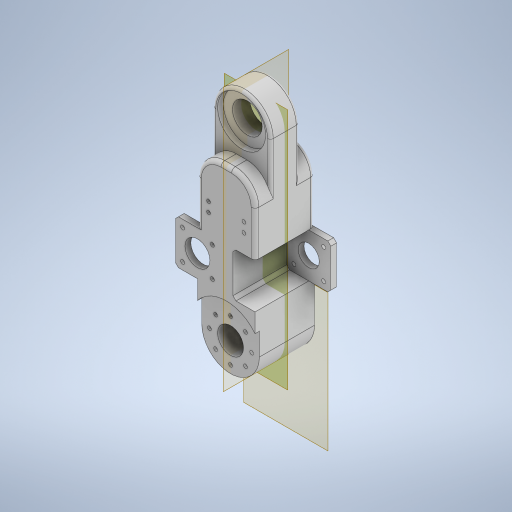
# Autodesk Inventor part: lower arm
Saved by Autodesk Inventor 2024 (Build 280153000, 153)
## iProperties
Created: 2024-02-21
Part Number: lower arm
Material: Generic
Document SubType Name: Modeling
Designer: MaartenGeorgesBuelen
Density: 1 g/cm^3
Appearance: Default
Author: MaartenGeorgesBuelen
## iProperties of the stored document lower arm_3DPrint.ipt
Created: 2024-02-21
Part Number: lower arm_3DPrint
Material: Generic
Document SubType Name: Modeling
Designer: MaartenGeorgesBuelen
Density: 1 g/cm^3
Appearance: Default
Author: MaartenGeorgesBuelen
Autodesk Inventor part; units mm, degrees
ref_plane "YZ Plane" through (0, 0, 0) normal (1, 0, 0) x (0, 1, 0)
ref_plane "XZ Plane" through (0, 0, 0) normal (0, 1, 0) x (-1, 0, 0)
ref_plane "Work Plane1" through (0, 0, 0) normal (0, 0, 1) x (1, 0, 0)
sketch "main" plane through (0, 0, 0) normal (0, 0, 1) x (1, 0, 0)
  circle A0 centre (35, 100) radius 13.5 projected
  arc A1 (31.5, 130) -> (0, 98.5) centre (31.5, 98.5) ccw projected
  line L0 (31.5, 130) -> (38.5, 130) projected
  arc A2 (70, 98.5) -> (38.5, 130) centre (38.5, 98.5) ccw projected
  circle A3 centre (35, 100) radius 30
  line L1 (5, 100) -> (65, 100)
  line L2 (65, 100) -> (65, 260)
  line L3 (65, 260) -> (5, 260)
  line L4 (5, 260) -> (5, 100)
  line L5 (55, 260) -> (15, 260)
  point P0 (0, 0)
  point P1 (0.0085, 99.2302)
  point P2 (69.9915, 99.2302)
  point P3 (35, 70)
  point P4 (48.5, 100)
  point P5 (21.5, 100)
  dimension "d0" = 60
  dimension "d4" = 160
  dimension "d5" = 60
  dimension "d6" = 30
  constraints: 10 end point, 2 horizontal, 2 parallel, 2 point on circle, 1 centre point, 1 coincident, 1 perpendicular, 1 point on line
  measures "d0" diameter of A3
  measures "d4" distance of L2.end L1.end
  measures "d5" distance of L2.end L3.end
  measures "d6" distance from line of A3.centre L4
ref_plane "Work Plane2" through (0, 68.4, 62) normal (0, 0, -1) x (0, 1, 0)
extrude "main extrude" add sketch "main" along normal up to surface (62 mm away) contours L1 A3 A0 | A0 L1 A3 | A3 L0 A2 L2 | L4 A1 L0 A3 | L0 A1 L4 L3 L2 A2
ref_plane "midplane" through (0, 0, 31) normal (0, 0, -1) x (-1, 0, 0)
mirror "right motor" about plane through (0, 0, 31) normal (0, 0, -1)
sketch "Sketch7" plane through (35, 100, 62) normal (0, 0, 1) x (1, 0, 0)
  circle A0 centre (-15.5563, 15.5563) radius 2
  circle A1 centre (0, 22) radius 2
  circle A2 centre (15.5563, 15.5563) radius 2
  circle A3 centre (22, 0) radius 2
  circle A4 centre (15.5563, -15.5563) radius 2
  circle A5 centre (0, -22) radius 2
  circle A6 centre (-15.5563, -15.5563) radius 2
  circle A7 centre (-22, 0) radius 2
  point P0 (-35, -100)
  constraints: 8 centre point, 16 other
extrude "screwholes" cut sketch "Sketch7" against normal blind 10
sketch "Sketch8" plane through (65, 100, 0) normal (1, 0, 0) x (0, 0, -1)
  line L0 (-62, 0) -> (-62, 160) projected
  line L1 (0, 0) -> (-62, 0) projected
  line L2 (0, 0) -> (0, 160) projected
  line L3 (0, 160) -> (-62, 160) projected
  line L4 (-31, 160) -> (-16, 160)
  line L5 (-16, 160) -> (-16, 220)
  line L6 (-16, 220) -> (-31, 220)
  line L7 (-31, 220) -> (-31, 160)
  line L8 (-31, 220) -> (-46, 220)
  line L9 (-46, 220) -> (-46, 160)
  line L10 (-46, 160) -> (-31, 160)
  line L11 (-31, 160) -> (-31, 220)
  point P0 (0, -100)
  point P1 (-46, 160)
  dimension "d39" = 15
  dimension "d40" = 60
  dimension "d41" = 15
  constraints: 16 end point, 5 parallel, 2 horizontal, 2 perpendicular, 1 midpoint
  measures "d39" distance of L6.end L5.end
  measures "d40" distance of L5.end L4.end
  measures "d41" distance of L10.end L9.end
extrude "arm joint" add sketch "Sketch8" against normal up to surface (60 mm away) contours L9 L8 L7 L3 | L7 L6 L5 L3
sketch "Sketch10" plane through (65, 260, 16) normal (0, 0, -1) x (-1, 0, 0)
  line L0 (60, 0) -> (60, 60) projected
  line L1 (0, 60) -> (60, 60) projected
  line L2 (0, 0) -> (0, 60) projected
  line L3 (60, 0) -> (0, 0) projected
  circle A0 centre (30, 32.1294) radius 19
  circle A1 centre (30, 32.1294) radius 13.5
  circle A2 centre (30, 32.1294) radius 25
  point P0 (65, -260)
  dimension "d93" = 4.2
  dimension "d45" = 38
  dimension "d46" = 27
  dimension "d47" = 6
  constraints: 3 centre point, 1 coincident
  measures "d45" diameter of A0
  measures "d46" diameter of A1
  measures "d47" radial gap between concentric circles of A0 A2
extrude "bearing hole" cut sketch "Sketch10" against normal blind 6 contours A0 | A1 | A2
sketch "Sketch11" plane through (35, 292.1294, 22) normal (0, 0, -1) x (-1, 0, 0)
  circle A0 centre (0, 0) radius 25 projected
  circle A1 centre (0, 0) radius 13.5
  point P0 (35, -292.1294)
  dimension "d50" = 27
  constraints: 1 centre point, 1 coincident
  measures "d50" diameter of A1
extrude "axle hole" cut sketch "Sketch11" against normal through all contours A1
mirror "Mirror3" about plane through (0, 0, 31) normal (0, 0, -1) of "bearing hole"
fillet "Fillet1" radius 30 2 edges at (65, 320, 31) (5, 320, 31)
fillet "Fillet3" radius 24.5 2 edges at (5, 260, 54) (65, 260, 54)
mirror "Mirror4" about plane through (0, 0, 31) normal (0, 0, -1) of "Fillet3"
sketch "Sketch14" plane through (35, 100, 62) normal (0, 0, 1) x (1, 0, 0)
  line L0 (9, 85) -> (11, 87) projected
  line L1 (9, 47) -> (9, 85) projected
  line L2 (11, 45) -> (9, 47) projected
  line L3 (49, 45) -> (11, 45) projected
  line L4 (51, 47) -> (49, 45) projected
  line L5 (51, 85) -> (51, 47) projected
  line L6 (49, 87) -> (51, 85) projected
  line L7 (11, 87) -> (49, 87) projected
  line L8 (49.8284, 89) -> (53, 85.8284)
  line L9 (53, 85.8284) -> (53, 46.1716)
  line L10 (53, 46.1716) -> (49.8284, 43)
  line L11 (49.8284, 43) -> (10.1716, 43)
  line L12 (10.1716, 43) -> (7, 46.1716)
  line L13 (7, 46.1716) -> (7, 85.8284)
  line L14 (7, 85.8284) -> (10.1716, 89)
  line L15 (10.1716, 89) -> (49.8284, 89)
  point P0 (-35, -100)
  dimension "d65" = 2
  constraints: 16 end point, 7 other
  measures "d65" distance between parallel lines of L7 L15
extrude "Extrusion12" cut sketch "Sketch14" against normal up to surface (62 mm away) contours L0 L7 L6 L5 L4 L3 L2 L1 | L8 L9 L10 L11 L12 L13 L14 L15
sketch "Sketch17" plane through (0, 0, 0) normal (0, 0, -1) x (-1, 0, 0)
  line L0 (16, 147) -> (14, 145) projected
  line L1 (16, 185) -> (16, 147) projected
  line L2 (14, 187) -> (16, 185) projected
  line L3 (-24, 187) -> (14, 187) projected
  line L4 (-26, 185) -> (-24, 187) projected
  line L5 (-26, 147) -> (-26, 185) projected
  line L6 (-24, 145) -> (-26, 147) projected
  line L7 (14, 145) -> (-24, 145) projected
  line L8 (14.8284, 189) -> (18, 185.8284)
  line L9 (18, 185.8284) -> (18, 146.1716)
  line L10 (18, 146.1716) -> (14.8284, 143)
  line L11 (14.8284, 143) -> (-24.8284, 143)
  line L12 (-24.8284, 143) -> (-28, 146.1716)
  line L13 (-28, 146.1716) -> (-28, 185.8284)
  line L14 (-28, 185.8284) -> (-24.8284, 189)
  line L15 (-24.8284, 189) -> (14.8284, 189)
  point P0 (0, 0)
  dimension "d72" = 2
  constraints: 16 end point, 7 other
  measures "d72" distance between parallel lines of L3 L15
extrude "Extrusion14" cut sketch "Sketch17" against normal up to surface (62 mm away) contours L0 L7 L6 L5 L4 L3 L2 L1 | L8 L9 L10 L11 L12 L13 L14 L15
sketch "Sketch18" plane through (35, 100, 62) normal (0, 0, 1) x (1, 0, 0)
  circle A0 centre (-14.5, 50.5) radius 1.5 projected
  circle A1 centre (-14.5, 81.5) radius 1.5 projected
  circle A2 centre (-45.5, 50.5) radius 1.5 projected
  circle A3 centre (-45.5, 81.5) radius 1.5 projected
  circle A4 centre (-30, 66) radius 11 projected
  line L0 (-49, 45) -> (-51, 47) projected
  line L1 (-49, 45) -> (-11, 45) projected
  line L2 (-9, 47) -> (-11, 45) projected
  line L3 (-9, 47) -> (-9, 85) projected
  line L4 (-11, 87) -> (-9, 85) projected
  line L5 (-11, 87) -> (-49, 87) projected
  line L6 (-51, 85) -> (-49, 87) projected
  line L7 (-51, 85) -> (-51, 47) projected
  line L8 (-49.8284, 89) -> (-10.1716, 89)
  line L9 (-10.1716, 89) -> (-7, 85.8284)
  line L10 (-7, 85.8284) -> (-7, 46.1716)
  line L11 (-7, 46.1716) -> (-10.1716, 43)
  line L12 (-10.1716, 43) -> (-49.8284, 43)
  line L13 (-49.8284, 43) -> (-53, 46.1716)
  line L14 (-53, 46.1716) -> (-53, 85.8284)
  line L15 (-53, 85.8284) -> (-49.8284, 89)
  circle A5 centre (-30, 66) radius 13
  circle A6 centre (-45.5, 81.5) radius 2.1
  circle A7 centre (-14.5, 81.5) radius 2.1
  circle A8 centre (-14.5, 50.5) radius 2.1
  circle A9 centre (-45.5, 50.5) radius 2.1
  point P0 (-35, -100)
  dimension "d84" = 2
  dimension "d85" = 2
  dimension "d86" = 4.2
  constraints: 16 end point, 5 centre point, 4 coincident, 3 equal radius, 7 other
  measures "d84" distance between parallel lines of L5 L8
  measures "d85" radial gap between concentric circles of A4 A5
  measures "d86" diameter of A6
extrude "Extrusion15" add sketch "Sketch18" against normal blind 6 contours L0 L7 L6 L5 L4 L3 L2 L1 | L8 L9 L10 L11 L12 L13 L14 L15
sketch "Sketch19" plane through (0, 0, 0) normal (0, 0, -1) x (-1, 0, 0)
  circle A0 centre (-80.5, 181.5) radius 1.5 projected
  circle A1 centre (-80.5, 150.5) radius 1.5 projected
  circle A2 centre (-49.5, 181.5) radius 1.5 projected
  circle A3 centre (-49.5, 150.5) radius 1.5 projected
  circle A4 centre (-65, 166) radius 11 projected
  line L0 (-46, 187) -> (-44, 185) projected
  line L1 (-46, 187) -> (-84, 187) projected
  line L2 (-86, 185) -> (-84, 187) projected
  line L3 (-86, 185) -> (-86, 147) projected
  line L4 (-84, 145) -> (-86, 147) projected
  line L5 (-84, 145) -> (-46, 145) projected
  line L6 (-44, 147) -> (-46, 145) projected
  line L7 (-44, 147) -> (-44, 185) projected
  line L8 (-84.8284, 189) -> (-45.1716, 189)
  line L9 (-45.1716, 189) -> (-42, 185.8284)
  line L10 (-42, 185.8284) -> (-42, 146.1716)
  line L11 (-42, 146.1716) -> (-45.1716, 143)
  line L12 (-45.1716, 143) -> (-84.8284, 143)
  line L13 (-84.8284, 143) -> (-88, 146.1716)
  line L14 (-88, 146.1716) -> (-88, 185.8284)
  line L15 (-88, 185.8284) -> (-84.8284, 189)
  circle A5 centre (-65, 166) radius 13
  circle A6 centre (-80.5, 181.5) radius 2.1
  circle A7 centre (-49.5, 181.5) radius 2.1
  circle A8 centre (-49.5, 150.5) radius 2.1
  circle A9 centre (-80.5, 150.5) radius 2.1
  point P0 (0, 0)
  dimension "d89" = 2
  dimension "d90" = 2
  dimension "d91" = 4.2
  dimension "d92" = 4.2
  dimension "d93" = 4.2
  dimension "d94" = 4.2
  constraints: 16 end point, 5 centre point, 4 coincident, 7 other
  measures "d89" distance between parallel lines of L1 L8
  measures "d90" radial gap between concentric circles of A4 A5
  measures "d91" diameter of A6
  measures "d92" diameter of A7
  measures "d93" diameter of A8
  measures "d94" diameter of A9
extrude "Extrusion16" add sketch "Sketch19" against normal blind 6 contours L0 L7 L6 L5 L4 L3 L2 L1 | L8 L9 L10 L11 L12 L13 L14 L15 | A5
fillet "Fillet5" radius 4 10 edges at (12.1759, 252.8241, 0) (35, 260, 0) (57.8241, 252.8241, 0) (65, 212.25, 0) (5, 212.25, 0) (12.1759, 252.8241, 62) (35, 260, 62) (57.8241, 252.8241, 62) (65, 212.25, 62) (5, 212.25, 62)
fillet "Fillet6" radius 3 10 edges at (13.7868, 311.2132, 16) (35, 320, 16) (56.2132, 311.2132, 16) (65, 262.75, 16) (5, 262.75, 16) (56.2132, 311.2132, 46) (35, 320, 46) (13.7868, 311.2132, 46) (65, 262.75, 46) (5, 262.75, 46)
fillet "Fillet7" [suppressed]
sketch "Sketch20" plane through (0, 0, 0) normal (0, 0, -1) x (-1, 0, 0)
  line L0 (-29.8752, 243.1601) -> (-29.8752, 192.4498) construction
  line L1 (-29.8752, 192.4498) -> (-44.0761, 192.4498) construction
  line L2 (-44.0761, 192.4498) -> (-44.0761, 243.1601) construction
  line L3 (-44.0761, 243.1601) -> (-29.8752, 243.1601) construction
  line L4 (-40.3367, 233.131) -> (-40.3367, 234.5213)
  line L5 (-40.3367, 234.5213) -> (-31.3249, 234.5213)
  line L6 (-31.3249, 234.5213) -> (-37.4543, 237.2511)
  line L7 (-37.4543, 237.2511) -> (-37.4543, 238.0989)
  line L8 (-37.4543, 238.0989) -> (-31.3249, 240.8033)
  line L9 (-31.3249, 240.8033) -> (-40.3367, 240.8033)
  line L10 (-40.3367, 240.8033) -> (-40.3367, 242.1004)
  line L11 (-40.3367, 242.1004) -> (-29.8752, 242.1004)
  line L12 (-29.8752, 242.1004) -> (-29.8752, 240.2014)
  line L13 (-29.8752, 240.2014) -> (-35.6994, 237.5903)
  line L14 (-35.6994, 237.5903) -> (-29.8752, 235.0639)
  line L15 (-29.8752, 235.0639) -> (-29.8752, 233.131)
  line L16 (-29.8752, 233.131) -> (-40.3367, 233.131)
  spline S0 degree 2 poles (-37.1236, 223.9157) (-37.9036, 223.9157) (-39.099, 224.5091) (-39.4889, 225.0008) knots 0 0 0 1 2 2 2
  spline S1 degree 2 poles (-39.4889, 225.0008) (-39.9467, 225.5943) (-40.3367, 226.9422) (-40.3367, 228.0104) knots 0 0 0 1 2 2 2
  line L17 (-40.3367, 228.0104) -> (-40.3367, 231.0115)
  line L18 (-40.3367, 231.0115) -> (-29.8752, 231.0115)
  line L19 (-29.8752, 231.0115) -> (-29.8752, 228.2393)
  spline S2 degree 2 poles (-29.8752, 228.2393) (-29.8752, 227.1203) (-30.0193, 226.0012) (-30.2991, 225.4926) knots 0 0 0 1 2 2 2
  spline S3 degree 2 poles (-30.2991, 225.4926) (-30.5958, 224.9245) (-31.5707, 224.4074) (-32.232, 224.4074) knots 0 0 0 1 2 2 2
  spline S4 degree 2 poles (-32.232, 224.4074) (-32.9696, 224.4074) (-34.1395, 225.1874) (-34.4701, 225.8741) knots 0 0 0 1 2 2 2
  line L20 (-34.4701, 225.8741) -> (-34.521, 225.8741)
  spline S5 degree 2 poles (-34.521, 225.8741) (-34.7753, 224.9415) (-36.1233, 223.9157) (-37.1236, 223.9157) knots 0 0 0 1 2 2 2
  spline S6 degree 2 poles (-37.183, 225.3654) (-36.5895, 225.3654) (-35.8266, 225.7045) (-35.5553, 226.2132) knots 0 0 0 1 2 2 2
  spline S7 degree 2 poles (-35.5553, 226.2132) (-35.3857, 226.5438) (-35.284, 227.3237) (-35.284, 228.0443) knots 0 0 0 1 2 2 2
  line L21 (-35.284, 228.0443) -> (-35.284, 229.6212)
  line L22 (-35.284, 229.6212) -> (-39.1498, 229.6212)
  line L23 (-39.1498, 229.6212) -> (-39.1498, 228.4937)
  spline S8 degree 2 poles (-39.1498, 228.4937) (-39.1498, 227.5781) (-38.9803, 226.5268) (-38.709, 226.1199) knots 0 0 0 1 2 2 2
  spline S9 degree 2 poles (-38.709, 226.1199) (-38.4292, 225.7299) (-37.734, 225.3654) (-37.183, 225.3654) knots 0 0 0 1 2 2 2
  spline S10 degree 2 poles (-32.427, 225.8571) (-32.054, 225.8571) (-31.4944, 226.1114) (-31.3334, 226.3912) knots 0 0 0 1 2 2 2
  spline S11 degree 2 poles (-31.3334, 226.3912) (-31.1469, 226.7303) (-31.0621, 227.5526) (-31.0621, 228.2902) knots 0 0 0 1 2 2 2
  line L24 (-31.0621, 228.2902) -> (-31.0621, 229.6212)
  line L25 (-31.0621, 229.6212) -> (-34.1225, 229.6212)
  line L26 (-34.1225, 229.6212) -> (-34.1225, 228.0443)
  spline S12 degree 2 poles (-34.1225, 228.0443) (-34.1225, 227.3916) (-33.9869, 226.7727) (-33.7749, 226.4421) knots 0 0 0 1 2 2 2
  spline S13 degree 2 poles (-33.7749, 226.4421) (-33.5715, 226.1199) (-32.9187, 225.8571) (-32.427, 225.8571) knots 0 0 0 1 2 2 2
  line L27 (-36.3946, 218.9986) -> (-36.3946, 222.9577)
  line L28 (-36.3946, 222.9577) -> (-35.1229, 222.9577)
  line L29 (-35.1229, 222.9577) -> (-35.1229, 218.9986)
  line L30 (-35.1229, 218.9986) -> (-36.3946, 218.9986)
  spline S14 degree 2 poles (-39.5059, 213.0388) (-39.6246, 213.1999) (-40.0485, 213.7424) (-40.1756, 213.9968) knots 0 0 0 1 2 2 2
  spline S15 degree 2 poles (-40.1756, 213.9968) (-40.3621, 214.3444) (-40.5571, 214.9971) (-40.5571, 215.5906) knots 0 0 0 1 2 2 2
  spline S16 degree 2 poles (-40.5571, 215.5906) (-40.5571, 216.0738) (-40.1926, 216.947) (-39.8619, 217.2776) knots 0 0 0 1 2 2 2
  spline S17 degree 2 poles (-39.8619, 217.2776) (-39.5398, 217.5913) (-38.5903, 217.9728) (-38.0647, 217.9728) knots 0 0 0 1 2 2 2
  spline S18 degree 2 poles (-38.0647, 217.9728) (-37.2508, 217.9728) (-36.0978, 217.2861) (-35.7672, 216.5401) knots 0 0 0 1 2 2 2
  spline S19 degree 2 poles (-35.7672, 216.5401) (-35.462, 215.8788) (-35.2331, 214.0815) (-35.1738, 213.0388) knots 0 0 0 1 2 2 2
  line L31 (-35.1738, 213.0388) -> (-34.9194, 213.0388)
  spline S20 degree 2 poles (-34.9194, 213.0388) (-34.4616, 213.0388) (-33.8936, 213.3186) (-33.7326, 213.5729) knots 0 0 0 1 2 2 2
  spline S21 degree 2 poles (-33.7326, 213.5729) (-33.5715, 213.8272) (-33.4698, 214.5563) (-33.4698, 214.9463) knots 0 0 0 1 2 2 2
  spline S22 degree 2 poles (-33.4698, 214.9463) (-33.4698, 215.4041) (-33.741, 216.6418) (-34.0038, 217.2607) knots 0 0 0 1 2 2 2
  line L32 (-34.0038, 217.2607) -> (-34.0038, 217.337)
  line L33 (-34.0038, 217.337) -> (-32.6559, 217.337)
  spline S23 degree 2 poles (-32.6559, 217.337) (-32.5542, 216.9724) (-32.2998, 215.6075) (-32.2998, 214.9378) knots 0 0 0 1 2 2 2
  spline S24 degree 2 poles (-32.2998, 214.9378) (-32.2998, 214.1239) (-32.5542, 213.0134) (-32.8848, 212.5725) knots 0 0 0 1 2 2 2
  spline S25 degree 2 poles (-32.8848, 212.5725) (-33.2069, 212.1402) (-34.2327, 211.7163) (-34.9703, 211.7163) knots 0 0 0 1 2 2 2
  line L34 (-34.9703, 211.7163) -> (-40.3367, 211.7163)
  line L35 (-40.3367, 211.7163) -> (-40.3367, 213.0388)
  line L36 (-40.3367, 213.0388) -> (-39.5059, 213.0388)
  line L37 (-38.4038, 213.0388) -> (-36.225, 213.0388)
  spline S26 degree 2 poles (-36.225, 213.0388) (-36.2674, 213.5135) (-36.4115, 214.9463) (-36.5472, 215.3956) knots 0 0 0 1 2 2 2
  spline S27 degree 2 poles (-36.5472, 215.3956) (-36.7082, 215.9212) (-37.378, 216.6079) (-37.9714, 216.6079) knots 0 0 0 1 2 2 2
  spline S28 degree 2 poles (-37.9714, 216.6079) (-38.6496, 216.6079) (-39.3363, 215.8449) (-39.3363, 215.1158) knots 0 0 0 1 2 2 2
  spline S29 degree 2 poles (-39.3363, 215.1158) (-39.3363, 214.497) (-38.8022, 213.4796) (-38.4038, 213.0388) knots 0 0 0 1 2 2 2
  line L38 (-33.9021, 205.6971) -> (-33.9021, 205.7649)
  spline S30 degree 2 poles (-33.9021, 205.7649) (-33.8597, 205.9175) (-33.8428, 206.2481) (-33.8428, 206.477) knots 0 0 0 1 2 2 2
  spline S31 degree 2 poles (-33.8428, 206.477) (-33.8428, 207.0111) (-34.309, 208.0624) (-34.7668, 208.5371) knots 0 0 0 1 2 2 2
  line L39 (-34.7668, 208.5371) -> (-40.3367, 208.5371)
  line L40 (-40.3367, 208.5371) -> (-40.3367, 209.8596)
  line L41 (-40.3367, 209.8596) -> (-32.4863, 209.8596)
  line L42 (-32.4863, 209.8596) -> (-32.4863, 208.5371)
  line L43 (-32.4863, 208.5371) -> (-33.6563, 208.5371)
  spline S32 degree 2 poles (-33.6563, 208.5371) (-33.012, 207.8165) (-32.4863, 206.7398) (-32.4863, 206.2312) knots 0 0 0 1 2 2 2
  spline S33 degree 2 poles (-32.4863, 206.2312) (-32.4863, 206.0277) (-32.5033, 205.8243) (-32.5287, 205.6971) knots 0 0 0 1 2 2 2
  line L44 (-32.5287, 205.6971) -> (-33.9021, 205.6971)
  line L45 (-40.3367, 195.7697) -> (-35.7926, 195.7697)
  spline S34 degree 2 poles (-35.7926, 195.7697) (-35.2501, 195.7697) (-34.326, 195.8545) (-34.0717, 195.9901) knots 0 0 0 1 2 2 2
  spline S35 degree 2 poles (-34.0717, 195.9901) (-33.7919, 196.1257) (-33.5206, 196.6429) (-33.5206, 197.0922) knots 0 0 0 1 2 2 2
  spline S36 degree 2 poles (-33.5206, 197.0922) (-33.5206, 197.4991) (-34.0208, 198.4317) (-34.4956, 198.9234) knots 0 0 0 1 2 2 2
  spline S37 degree 2 poles (-34.4956, 198.9234) (-34.6142, 198.9149) (-34.9449, 198.898) (-35.1653, 198.898) knots 0 0 0 1 2 2 2
  line L46 (-35.1653, 198.898) -> (-40.3367, 198.898)
  line L47 (-40.3367, 198.898) -> (-40.3367, 200.2205)
  line L48 (-40.3367, 200.2205) -> (-35.7926, 200.2205)
  spline S38 degree 2 poles (-35.7926, 200.2205) (-35.2501, 200.2205) (-34.326, 200.3053) (-34.0717, 200.4409) knots 0 0 0 1 2 2 2
  spline S39 degree 2 poles (-34.0717, 200.4409) (-33.7919, 200.5765) (-33.5206, 201.0937) (-33.5206, 201.543) knots 0 0 0 1 2 2 2
  spline S40 degree 2 poles (-33.5206, 201.543) (-33.5206, 201.9669) (-34.0547, 202.9079) (-34.4701, 203.3488) knots 0 0 0 1 2 2 2
  line L49 (-34.4701, 203.3488) -> (-40.3367, 203.3488)
  line L50 (-40.3367, 203.3488) -> (-40.3367, 204.6713)
  line L51 (-40.3367, 204.6713) -> (-32.4863, 204.6713)
  line L52 (-32.4863, 204.6713) -> (-32.4863, 203.3488)
  line L53 (-32.4863, 203.3488) -> (-33.3511, 203.3488)
  spline S41 degree 2 poles (-33.3511, 203.3488) (-32.8339, 202.8316) (-32.2659, 201.8143) (-32.2659, 201.2039) knots 0 0 0 1 2 2 2
  spline S42 degree 2 poles (-32.2659, 201.2039) (-32.2659, 200.5087) (-32.9017, 199.4321) (-33.6223, 199.1523) knots 0 0 0 1 2 2 2
  spline S43 degree 2 poles (-33.6223, 199.1523) (-32.9526, 198.5504) (-32.2659, 197.4144) (-32.2659, 196.7531) knots 0 0 0 1 2 2 2
  spline S44 degree 2 poles (-32.2659, 196.7531) (-32.2659, 196.2444) (-32.5796, 195.4136) (-32.9357, 195.1084) knots 0 0 0 1 2 2 2
  spline S45 degree 2 poles (-32.9357, 195.1084) (-33.2917, 194.7947) (-34.3599, 194.4472) (-35.1653, 194.4472) knots 0 0 0 1 2 2 2
  line L54 (-35.1653, 194.4472) -> (-40.3367, 194.4472)
  line L55 (-40.3367, 194.4472) -> (-40.3367, 195.7697)
  point P0 (0, 0)
  constraints: 2 other
extrude "Extrusion17" cut sketch "Sketch20" against normal blind 1
sketch "Sketch21" plane through (0, 0, 0) normal (0, 0, -1) x (-1, 0, 0)
  circle A0 centre (-53.4345, 208.6439) radius 1.95
  circle A1 centre (-53.4345, 218.6439) radius 1.95
  line L0 (-29.5, 260) -> (-40.5, 260) projected
  line L1 (-65, 235.5) -> (-65, 189) projected
  point P0 (0, 0)
  point P1 (-35, 260)
  dimension "d102" = 3.9
  dimension "d103" = 3.9
  dimension "d104" = 10
  dimension "d105" = 45.2787
  dimension "d106" = 11.5655
  constraints: 2 centre point, 1 midpoint
  measures "d102" diameter of A0
  measures "d103" diameter of A1
  measures "d104" distance of A1.centre A0.centre
  measures "d105" distance of point (-35, 260) A1.centre
  measures "d106" distance from line of L1 A1.centre
extrude "Extrusion18" cut sketch "Sketch21" against normal through all
sketch "Sketch22" plane through (35, 100, 62) normal (0, 0, 1) x (1, 0, 0)
  circle A0 centre (0, 0) radius 30
  circle A1 centre (0, 0) radius 38
  point P0 (-35, -100)
  dimension "d109" = 8
  constraints: 2 centre point, 2 other
  measures "d109" radial gap between concentric circles of A0 A1
extrude "Extrusion19" cut sketch "Sketch22" against normal blind 4.5 contours A0 | A1
ref_plane "Work Plane6" through (35, 189, 58) normal (1, 0, 0) x (0, 0, -1)
mirror "Mirror5" about plane through (35, 189, 58) normal (1, 0, 0) of "Extrusion18"
sketch "Sketch23" plane through (35, 292.1294, 22) normal (0, 0, -1) x (-1, 0, 0)
  circle A0 centre (0, 0) radius 13.5 projected
  circle A1 centre (0, 0) radius 25 projected
  circle A2 centre (0, 0) radius 15.5
  point P0 (35, -292.1294)
  dimension "d112" = 2
  constraints: 1 centre point
  measures "d112" radial gap between concentric circles of A0 A2
extrude "Extrusion20" cut sketch "Sketch23" against normal through all contours A0 | A2
ref_plane "Work Plane5" through (0, 0, 31) normal (0, 0, -1) x (-1, 0, 0)
equation "\"d4\" = main_length"
equation "\"main_length\" = 160"
body "Solid1"
